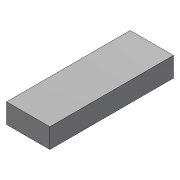
# Autodesk Inventor part: BLANK-BC-10001
Saved by Autodesk Inventor 2016 (Build 200138000, 138)
## iProperties
Created: 2015-12-02
Part Number: BLANK-BC-10001
Project: DIPOLO BC-3T- SIRIUS
Cost Center: 1504002005
Material: Aço Carbono
Document SubType Name: Modeling
Designer: reinaldo.basilio
Density: 7.87 g/cm^3
Appearance: Aço(1)
Mass: 395258 g
Surface Area: 10232.5 cm^2
Volume: 50223.4 cm^3
Description: Base de referência de montagem do BC.
RuleStatus: InUse
AfterMaterialChange0: file://_iMaterial
AfterAnyiPropertyChange0: file://_iMaterial
AfterDocNew0: file://_Naming_par
AfterDocNew1: file://_NameStart
AfterDocNew2: file://_NameStart1
AfterDocNew3: file://_Materiais
DocNumber: XXXXX-XXX-XXXX-00-001.ipt
Folder: .
Title: DIPOLO BC-3T- SIRIUS
Author: reinaldo.basilio
Subject: BLANK-BC-10001
Autodesk Inventor part; units mm, degrees
ref_plane "YZ Plane" through (0, 0, 0) normal (1, 0, 0) x (0, 1, 0)
ref_plane "XZ Plane" through (0, 0, 0) normal (0, 1, 0) x (-1, 0, 0)
ref_plane "XY Plane" through (0, 0, 0) normal (0, 0, 1) x (1, 0, 0)
sketch "Sketch5" plane through (0, 0, 0) normal (0, 0, 1) x (1, 0, 0)
  line L0 (-461.5, 161.5) -> (461.5, 161.5)
  line L1 (461.5, 161.5) -> (461.5, -161.5)
  line L2 (461.5, -161.5) -> (-461.5, -161.5)
  line L3 (-461.5, -161.5) -> (-461.5, 161.5)
  point P0 (0, 0)
  point P1 (0, 161.5)
  point P2 (-461.5, 0)
  dimension "d8" = 923
  dimension "d164" = 323
  constraints: 8 end point, 2 midpoint, 2 parallel, 1 horizontal, 1 horizontal alignment, 1 perpendicular, 1 vertical alignment
  measures "d8" distance of L0.start L0.end
  measures "d164" distance of L2.end L0.start
extrude "Extrusion5" add sketch "Sketch5" along normal blind 147.5
body "Solid5"
